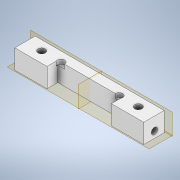
# Autodesk Inventor part: Fuehrungslagerhalter_v2
Saved by Autodesk Inventor 2022 (Build 260153000, 153)
## iProperties
Created: 2022-04-21
Part Number: Fuehrungslagerhalter_v2
Material: PBT-Kunststoff
Document SubType Name: Modeling
Designer: 123St
Density: 1.31 g/cm^3
Appearance: Glatt - Weiß
Mass: 4.68181 g
Surface Area: 25.9083 cm^2
Volume: 3.5739 cm^3
Author: 123St
Autodesk Inventor part; units mm, degrees
sketch "Skizze1" plane through (0, 0, 0) normal (0, 1, 0) x (-1, 0, 0)
  line L0 (30, 0.2989) -> (30, 10.2989)
  line L1 (30, 10.2989) -> (15, 10.2989)
  line L2 (15, 10.2989) -> (15, 5.2989)
  line L3 (15, 5.2989) -> (-15, 5.2989)
  line L4 (-15, 5.2989) -> (-15, 10.2989)
  line L5 (-15, 10.2989) -> (-30, 10.2989)
  line L6 (-30, 10.2989) -> (-30, 0.2989)
  line L7 (-30, 0.2989) -> (30, 0.2989)
  line L8 (0, -2.0598) -> (0, 12.3587) projected
  point P0 (0, 0)
  dimension "d0" = 30
  dimension "d1" = 5
  dimension "d2" = 15
  dimension "d3" = 15
  dimension "d4" = 15
  dimension "d5" = 5
  constraints: 16 end point, 6 perpendicular, 2 point on line, 1 vertical
  measures "d0" distance of L2.end L3.end
  measures "d1" distance of L1.end L2.end
  measures "d2" distance between parallel lines of L8 L4
  measures "d3" distance of L0.end L1.end
  measures "d4" distance of L4.end L5.end
  measures "d5" distance between parallel lines of L3 L7
extrude "Extrusion1" add sketch "Skizze1" along normal blind 9
sketch "Skizze2" plane through (30, 0, 10.2989) normal (1, 0, 0) x (0, 0, -1)
  circle A0 centre (5, 3) radius 1.5
  line L0 (0, 0) -> (0, 9) construction
  line L1 (0, 0) -> (10, 0) construction
  point P0 (10.2989, 0)
  dimension "d8" = 3
  dimension "d9" = 5
  dimension "d43" = 3
  dimension "d60" = 9
  dimension "d61" = 10
  constraints: 1 centre point
  measures "d8" diameter of A0
  measures "d9" distance from line of L0 A0.centre
  measures "d43" distance from line of L1 A0.centre
  measures "d60" distance from line of L0.end L1
  measures "d61" distance of L0.start L1.end
extrude "Extrusion2" cut sketch "Skizze2" against normal blind 4
sketch "Skizze4" plane through (-30, 0, 0.2989) normal (-1, 0, 0) x (0, 0, 1)
  circle A0 centre (5, 3) radius 1.5 projected
  circle A1 centre (5, 3) radius 1.5
  line L0 (10, 0) -> (10, 9) projected
  line L1 (0, 0) -> (10, 0) projected
  point P0 (-0.2989, 0)
  dimension "d21" = 5
  dimension "d22" = 3
  dimension "d63" = 3
  constraints: 1 centre point, 1 coincident
  measures "d21" distance from line of L0 A1.centre
  measures "d22" distance from line of L1 A1.centre
  measures "d63" diameter of A1
extrude "Extrusion4" cut sketch "Skizze4" against normal blind 4
sketch "Skizze5" plane through (0, 0, 0) normal (0, 1, 0) x (1, 0, 0)
  circle A0 centre (-22.5, -5.2989) radius 1.5
  circle A1 centre (22.5, -5.2989) radius 1.5
  line L0 (-30, -10.2989) -> (-15, -10.2989) projected
  line L1 (-30, -0.2989) -> (-30, -10.2989) projected
  line L2 (30, -10.2989) -> (30, -0.2989) projected
  line L3 (15, -10.2989) -> (30, -10.2989) projected
  point P0 (0, 0)
  dimension "d25" = 5
  dimension "d26" = 7.5
  dimension "d27" = 7.5
  dimension "d28" = 5
  dimension "d29" = 3
  dimension "d30" = 3
  constraints: 2 centre point, 2 coincident
  measures "d25" distance from line of L0 A0.centre
  measures "d26" distance from line of L1 A0.centre
  measures "d27" distance from line of L2 A1.centre
  measures "d28" distance from line of L3 A1.centre
  measures "d29" diameter of A0
  measures "d30" diameter of A1
hole "Bohrung1" at (-22.5, 0, 5.2989) at (22.5, 0, 5.2989) direction (0, 1, 0) diameter 3.4 end through all counterbore diameter 6.5 counterbore depth 3.4 clearance for "Inbusschraube DIN EN ISO 4762" size "M3" standard "DIN"
sketch "Skizze6" plane through (0, 0, 0) normal (0, -1, 0) x (1, 0, 0)
  circle A0 centre (-7, 2.7989) radius 1.5
  circle A1 centre (7, 2.7989) radius 1.5
  line L0 (-30, 0.2989) -> (-30, 10.2989) projected
  line L1 (-30, 10.2989) -> (-15, 10.2989) projected
  line L2 (15, 10.2989) -> (30, 10.2989) projected
  line L3 (30, 10.2989) -> (30, 0.2989) projected
  point P0 (0, 0)
  dimension "d33" = 3
  dimension "d34" = 3
  dimension "d36" = 7.5
  dimension "d37" = 7.5
  dimension "d41" = 7
  dimension "d42" = 7
  constraints: 2 centre point
  measures "d33" diameter of A1
  measures "d34" diameter of A0
  measures "d36" distance from line of L1 A0.centre
  measures "d37" distance from line of L2 A1.centre
  measures "d41" horizontal distance of point (0, 0) A0.centre
  measures "d42" horizontal distance of point (0, 0) A1.centre
extrude "Extrusion6" cut sketch "Skizze6" against normal blind 4
sketch "Skizze8" plane through (0, 9, 0) normal (0, 1, 0) x (1, 0, 0)
  circle A0 centre (-13.5, -5.2989) radius 1.7 projected
  circle A1 centre (13.5, -5.2989) radius 1.7 projected
  point P0 (0, 0)
extrude "Extrusion8" cut sketch "Skizze8" against normal blind 2
chamfer "Fase1" distance 0.5 angle 45 4 edges at (-30, 4.5, 0.2989) (0, 0, 0.2989) (0, 9, 0.2989) (30, 4.5, 0.2989)
equation "\"d2\" = 0.5 * d0"
equation "\"d9\" = 0.5 * d61"
equation "\"d33\" = d34"
equation "\"d42\" = d41"
